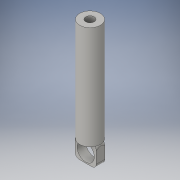
# Autodesk Inventor part: cylendar2
Saved by Autodesk Inventor 2016 (Build 200138000, 138)
## iProperties
Created: 2018-01-12
Part Number: cylendar2
Material: Generic
Document SubType Name: Modeling
Designer: New User
Density: 1 g/cm^3
Appearance: Default
Author: New User
Autodesk Inventor part; units mm, degrees
ref_plane "YZ Plane" through (0, 0, 0) normal (1, 0, 0) x (0, 1, 0)
ref_plane "XZ Plane" through (0, 0, 0) normal (0, 1, 0) x (-1, 0, 0)
ref_plane "XY Plane" through (0, 0, 0) normal (0, 0, 1) x (1, 0, 0)
sketch "Sketch1" plane through (0, 0, 0) normal (0, 1, 0) x (-1, 0, 0)
  circle A0 centre (0, 0) radius 3.81
  dimension "d0" = 7.62
  constraints: 1 centre point, 1 coincident
  measures "d0" diameter of A0
extrude "Extrusion1" add sketch "Sketch1" along normal blind 38.1
sketch "Sketch2" plane through (0, 38.1, 0) normal (0, 1, 0) x (1, 0, 0)
  circle A0 centre (0, 0) radius 1.5875
  dimension "d3" = 3.175
  constraints: 1 centre point, 1 coincident
  measures "d3" diameter of A0
extrude "Extrusion2" cut sketch "Sketch2" against normal blind 36.5125
sketch "Sketch3" plane through (0, 0, 0) normal (0, -1, 0) x (1, 0, 0)
  line L0 (3.8861, -1.5875) -> (-3.8861, -1.5875)
  line L1 (-3.8861, -1.5875) -> (-3.8861, 1.5875)
  line L2 (-3.8861, 1.5875) -> (3.8861, 1.5875)
  line L3 (3.8861, 1.5875) -> (3.8861, -1.5875)
  line L4 (3.8861, -1.5875) -> (-3.8861, 1.5875) construction
  line L5 (-3.8861, -1.5875) -> (3.8861, 1.5875) construction
  point P0 (0, 0)
  constraints: 12 end point, 2 midpoint, 2 parallel, 1 horizontal, 1 perpendicular
extrude "Extrusion3" add sketch "Sketch3" along normal blind 7.112
sketch "Sketch5" plane through (-3.8861, 0, 1.5875) normal (0, 0, 1) x (1, 0, 0)
  circle A0 centre (3.8861, -3.5629) radius 3.175
  point P0 (3.8861, 0)
  dimension "d16" = 6.35
  constraints: 1 centre point
  measures "d16" diameter of A0
extrude "Extrusion4" cut sketch "Sketch5" against normal blind 6.35
fillet "Fillet2" radius 1.5875 4 edges at (3.8861, 0, 0) (3.8861, -7.112, 0) (-3.8861, 0, 0) (-3.8861, -7.112, 0)
body "Solid1"
